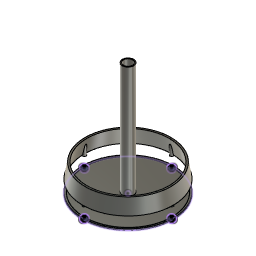
2022_10_18_VerticalScultureHolder v4 (Autodesk Fusion 360 design; units mm, degrees)
Autodesk Fusion 360 part; units mm, degrees
note: some values were not read from the file. Chosen so that the rebuilt part matches the saved one: a direction; which face or edge a step refers to; which pieces of a blend or face edit are solid. Set by a fixed rule: which sketch regions a step uses.
sketch "CircleSketch" plane through (0, 0, 0) normal (0, 0, 1) x (1, 0, 0)
  circle A0 centre (0, 0) radius 38.5
  circle A1 centre (0, 0) radius 40
  circle A2 centre (0, 0) radius 5
  circle A3 centre (0, 0) radius 4.1
  dimension "d6" = 80
  dimension "d7" = 10
  constraint coincident A0.centre A1.centre
  constraint concentric A0 A1
  constraint concentric A0 A2
  constraint concentric A2 A3
  measures "d6" diameter of A1
  measures "d7" diameter of A2
extrude "Extrude1" add sketch "CircleSketch" along normal blind 1.2 contours A0 | A1 | A2 | A3 makes body 1
extrude "Extrude2" add sketch "CircleSketch" along normal blind 10 contours A2 | A3 bodies 1
extrude "Extrude3" add sketch "CircleSketch" along normal blind 100 contours A2 bodies 1
sketch "Sketch2" plane through (0, 0, 0) normal (0, 1, 0) x (1, 0, 0)
extrude "Extrude4" add sketch "CircleSketch" along normal blind 13 separate body contours A1 makes body 2
sketch "Sketch3" plane through (0, 0, 0) normal (0, 0, 1) x (1, 0, 0)
  circle A0 centre (0, 0) radius 40
  circle A1 centre (0, 0) radius 40
  line L0 (0, 0) -> (40, 0)
  line L1 (0, 0) -> (0, 40)
  line L2 (0, 0) -> (0, -40)
  circle A2 centre (38.5, 0) radius 1.5
  circle A3 centre (0, 38.5) radius 1.5
  circle A4 centre (0, -38.5) radius 1.5
  line L3 (0, 0) -> (-38.5, 0)
  circle A5 centre (-38.5, 0) radius 1.5
  dimension "d37" = 80
  dimension "d38" = 40
  dimension "d39" = 40
  dimension "d40" = 40
  dimension "d42" = 3
  dimension "d43" = 3
  dimension "d44" = 3
  dimension "d46" = 38.5
  dimension "d47" = 3
  constraint coincident A0.centre A1.centre
  constraint horizontal L0
  constraint vertical L1
  constraint perpendicular L0 L2
  constraint coincident L0.end A2
  constraint coincident L1.end A3
  constraint coincident L2.end A4
  constraint perpendicular L2 L3
  constraint coincident L3.end A5.centre
  measures "d37" diameter of A0
  measures "d38" distance of A0.centre L0.end
  measures "d39" distance of A0.centre L1.end
  measures "d40" distance of A0.centre L2.end
  measures "d42" diameter of A2
  measures "d43" diameter of A3
  measures "d44" diameter of A4
  measures "d46" distance of A0.centre L3.end
  measures "d47" diameter of A5
extrude "Extrude5" add sketch "Sketch3" along normal blind 9 separate body contours L0 A2 | L0 A2 | L1 A3 | L1 A3 | L2 A4 | L2 A4 | A5 makes body 3 at (37.8157, 1.3348, 6) makes body 4 at (1.4095, 37.987, 3) makes body 5 at (-39.1843, 1.3348, 6) makes body 6 at (1.4095, -39.013, 3)
move_body "Move1" bodies 2 to x (1, 0, 0) y (0, 1, 0) z (0, 0, 1) at (0, 0, 1)
combine "Combine3" operation add target body 2 tool bodies 6 5 4 3
draft "Draft3" angle 10 neutral plane through (0, 0, 1) pull (0, 0, -1) 1 faces at (-5.7738, -38.0646, 8) on bodies 2
draft "Draft4" angle -10 neutral plane through (0, 0, 1) pull (0, 0, -1) 1 faces at (0, -40, 9.6667) on bodies 2
combine "Combine2" operation cut target body 1 tool bodies 2 keep tools
sketch "Sketch4" plane through (0, 0, 0) normal (0, 0, -1) x (1, 0, 0)
  circle A0 centre (-38.5, 0) radius 1.7
  circle A1 centre (0, 38.5) radius 1.7
  circle A2 centre (0, -38.5) radius 1.7
  circle A3 centre (38.5, 0) radius 1.7
  arc A4 (0, 40) -> (-40, 0) centre (0, 0) ccw
  circle A5 centre (-38.5, 0) radius 1.5
  arc A6 (-40, 0) -> (0, -40) centre (0, 0) ccw
  circle A7 centre (0, -38.5) radius 1.5
  arc A8 (0, -40) -> (40, 0) centre (0, 0) ccw
  circle A9 centre (38.5, 0) radius 1.5
  arc A10 (40, 0) -> (0, 40) centre (0, 0) ccw
  circle A11 centre (0, 38.5) radius 1.5
  point P0 (0, -38.5)
  point P1 (-38.5, 0)
  point P2 (0, 38.5)
  point P3 (38.5, 0)
  constraint coincident P0 A2.centre
  constraint coincident A0.centre A5.centre
  constraint coincident A1.centre A11.centre
  constraint coincident P3 A3.centre
extrude "Extrude6" cut sketch "Sketch3" sketch "Sketch4" against normal blind 60 contours L0 A2 | L0 A2 | L1 A3 | L1 A3 | L2 A4 | L2 A4 | A5 of sketch 2 contours A0 A4 A6 | A1 A4 A10 | A2 A6 A8 | A3 A8 A10 picked at (-39.8625, 0.895) picked at (-0.8905, 39.8656) picked at (-0.8905, -39.8656) picked at (39.8625, -0.895) bodies 1
sketch "Sketch5" plane through (0, 0, 0) normal (0, 1, 0) x (1, 0, 0)
move_body "Move2" bodies 2 to x (1, 0, 0) y (0, 1, 0) z (0, 0, 1) at (0, 0, 10)
equation "Dimension = 80 mm"
equation "BorderSize = 3 mm"
equation "InnerDiameter = 10 mm"
equation "InnerBorder = 1.8 mm"
equation "d5 = ( Dimension - BorderSize )"
equation "d6 = Dimension"
equation "d7 = InnerDiameter"
equation "d8 = ( InnerDiameter - InnerBorder )"
equation "PlateHeight = 2 mm"
equation "PlateJoinHeight = 10 mm"
equation "TubeHeight = 100 mm"
equation "d14 = PlateJoinHeight"
equation "d16 = TubeHeight"
equation "d18 = HeightOfStuffHolder"
equation "d20 = PlateHeight + 7 mm"
equation "HeightOfStuffHolder = 13 mm"
equation "d37 = Dimension"
equation "d38 = Dimension / 2"
equation "d39 = Dimension / 2"
equation "d40 = Dimension / 2"
equation "d42 = BorderSize"
equation "d43 = BorderSize"
equation "d44 = BorderSize"
equation "d46 = ( Dimension - BorderSize ) / 2"
equation "d47 = BorderSize"
named bodies: "ScultureHolder", "WeighHolder"
